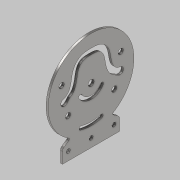
# Autodesk Inventor part: RR-PCSS-2021-W2M2MA2
Saved by Autodesk Inventor 2021 (Build 250183000, 183)
## iProperties
Created: 2021-10-12
Part Number: RR-PCSS-2021-W2M2MA2
Material: Stal nierdzewna
Document SubType Name: Konstrukcja blachowa
Designer: marci
Density: 8 g/cm^3
Sheet Metal Rule: Domyślny_mm
Appearance: Częściowo polerowana
Author: marci
Autodesk Inventor part; units mm, degrees
ref_plane "YZ Plane" through (0, 0, 0) normal (1, 0, 0) x (0, 1, 0)
ref_plane "XZ Plane" through (0, 0, 0) normal (0, 1, 0) x (-1, 0, 0)
ref_plane "XY Plane" through (0, 0, 0) normal (0, 0, 1) x (1, 0, 0)
sketch "Szkic1" plane through (0, 0, 0) normal (1, 0, 0) x (0, 1, 0)
  arc A0 (305.2016, 165.6304) -> (305.2016, 131.3696) centre (315.5238, 148.5) ccw
  arc A1 (307.7821, 161.3478) -> (305.2016, 165.6304) centre (306.4918, 163.4891) ccw
  arc A2 (307.7821, 161.3478) -> (307.7821, 135.6522) centre (315.5238, 148.5) ccw
  arc A3 (305.2016, 131.3696) -> (307.7821, 135.6522) centre (306.4918, 133.5109) ccw
  circle A4 centre (292.0124, 180.8607) radius 3.65
  circle A5 centre (333.1067, 189.9227) radius 3.65
  circle A6 centre (333.1067, 107.0773) radius 3.65
  circle A7 centre (292.0124, 116.1393) radius 3.65
  arc A8 (265.7342, 133.5) -> (270.5217, 134.9423) centre (268.128, 134.2212) ccw
  arc A9 (265.7342, 163.5) -> (265.7342, 133.5) centre (315.5238, 148.5) ccw
  arc A10 (270.5217, 162.0577) -> (265.7342, 163.5) centre (268.128, 162.7788) ccw
  arc A11 (270.5217, 162.0577) -> (270.5217, 134.9423) centre (315.5238, 148.5) ccw
  spline S0 degree 3 poles (357.7316, 148.5) (357.7316, 153.1999) (357.4798, 157.3219) (355.4595, 163.5199) (354.2505, 165.5182) (351.0648, 169.1973) (348.9327, 170.8743) (343.9224, 173.7031) (341.1419, 174.5841) (332.899, 176.2956) (327.9871, 176.7072) (321.7354, 179.3107) (319.9473, 180.4312) (317.422, 182.9628) (316.5959, 184.0618) (315.07, 186.6603) (315.3905, 188.1626) (314.1922, 189.4328) knots -9.163844 -9.163844 -9.163844 -9.163844 -7.753869 -7.753869 -6.746587 -6.746587 -5.59383 -5.59383 -4.201497 -4.201497 -2.238429 -2.238429 -1.297056 -1.297056 -0.700858 -0.700858 0 0 0 0
  line L0 (357.7316, 148.5) -> (357.7316, 153.1999) construction
  line L1 (357.7316, 153.1999) -> (357.4798, 157.3219) construction
  line L2 (357.4798, 157.3219) -> (355.4595, 163.5199) construction
  line L3 (355.4595, 163.5199) -> (354.2505, 165.5182) construction
  line L4 (354.2505, 165.5182) -> (351.0648, 169.1973) construction
  line L5 (351.0648, 169.1973) -> (348.9327, 170.8743) construction
  line L6 (348.9327, 170.8743) -> (343.9224, 173.7031) construction
  line L7 (343.9224, 173.7031) -> (341.1419, 174.5841) construction
  line L8 (341.1419, 174.5841) -> (332.899, 176.2956) construction
  line L9 (332.899, 176.2956) -> (327.9871, 176.7072) construction
  line L10 (327.9871, 176.7072) -> (321.7354, 179.3107) construction
  line L11 (321.7354, 179.3107) -> (319.9473, 180.4312) construction
  line L12 (319.9473, 180.4312) -> (317.422, 182.9628) construction
  line L13 (317.422, 182.9628) -> (316.5959, 184.0618) construction
  line L14 (316.5959, 184.0618) -> (315.07, 186.6603) construction
  line L15 (315.07, 186.6603) -> (315.3905, 188.1626) construction
  line L16 (315.3905, 188.1626) -> (314.1922, 189.4328) construction
  spline S1 degree 3 poles (314.7636, 107.2836) (315.1895, 110.0737) (316.0926, 112.3675) (318.7997, 115.5706) (320.2643, 116.7452) (323.9682, 118.7687) (326.1559, 119.4488) (333.914, 121.2316) (340.1639, 121.52) (348.3717, 125.6837) (350.9092, 127.5926) (354.3009, 131.5638) (355.4987, 133.5584) (357.4842, 139.7513) (357.7316, 143.8417) (357.7316, 148.5) knots -7.999364 -7.999364 -7.999364 -7.999364 -7.089801 -7.089801 -6.306276 -6.306276 -5.390174 -5.390174 -3.08524 -3.08524 -1.97401 -1.97401 -1.144907 -1.144907 0 0 0 0
  line L17 (314.7636, 107.2836) -> (315.1895, 110.0737) construction
  line L18 (315.1895, 110.0737) -> (316.0926, 112.3675) construction
  line L19 (316.0926, 112.3675) -> (318.7997, 115.5706) construction
  line L20 (318.7997, 115.5706) -> (320.2643, 116.7452) construction
  line L21 (320.2643, 116.7452) -> (323.9682, 118.7687) construction
  line L22 (323.9682, 118.7687) -> (326.1559, 119.4488) construction
  line L23 (326.1559, 119.4488) -> (333.914, 121.2316) construction
  line L24 (333.914, 121.2316) -> (340.1639, 121.52) construction
  line L25 (340.1639, 121.52) -> (348.3717, 125.6837) construction
  line L26 (348.3717, 125.6837) -> (350.9092, 127.5926) construction
  line L27 (350.9092, 127.5926) -> (354.3009, 131.5638) construction
  line L28 (354.3009, 131.5638) -> (355.4987, 133.5584) construction
  line L29 (355.4987, 133.5584) -> (357.4842, 139.7513) construction
  line L30 (357.4842, 139.7513) -> (357.7316, 143.8417) construction
  line L31 (357.7316, 143.8417) -> (357.7316, 148.5) construction
  arc A12 (305.7086, 110.17) -> (314.7636, 107.2836) centre (310.0075, 108.0096) ccw
  spline S2 degree 3 poles (349.7316, 148.5) (349.7316, 144.263) (349.5035, 141.031) (348.232, 137.1168) (347.6126, 136.0385) (345.6418, 133.7599) (344.2226, 132.6472) (340.9385, 130.8081) (339.0257, 130.1351) (331.2404, 128.5496) (325.7415, 128.0559) (318.2028, 124.8703) (315.3125, 123.2792) (311.2172, 119.1288) (309.9943, 117.5052) (307.7133, 113.5974) (306.4514, 111.648) (305.7086, 110.17) knots -6.764215 -6.764215 -6.764215 -6.764215 -5.493128 -5.493128 -4.764431 -4.764431 -3.885162 -3.885162 -2.898584 -2.898584 -1.437025 -1.437025 -0.780111 -0.780111 -0.427062 -0.427062 0 0 0 0
  line L32 (349.7316, 148.5) -> (349.7316, 144.263) construction
  line L33 (349.7316, 144.263) -> (349.5035, 141.031) construction
  line L34 (349.5035, 141.031) -> (348.232, 137.1168) construction
  line L35 (348.232, 137.1168) -> (347.6126, 136.0385) construction
  line L36 (347.6126, 136.0385) -> (345.6418, 133.7599) construction
  line L37 (345.6418, 133.7599) -> (344.2226, 132.6472) construction
  line L38 (344.2226, 132.6472) -> (340.9385, 130.8081) construction
  line L39 (340.9385, 130.8081) -> (339.0257, 130.1351) construction
  line L40 (339.0257, 130.1351) -> (331.2404, 128.5496) construction
  line L41 (331.2404, 128.5496) -> (325.7415, 128.0559) construction
  line L42 (325.7415, 128.0559) -> (318.2028, 124.8703) construction
  line L43 (318.2028, 124.8703) -> (315.3125, 123.2792) construction
  line L44 (315.3125, 123.2792) -> (311.2172, 119.1288) construction
  line L45 (311.2172, 119.1288) -> (309.9943, 117.5052) construction
  line L46 (309.9943, 117.5052) -> (307.7133, 113.5974) construction
  line L47 (307.7133, 113.5974) -> (306.4514, 111.648) construction
  line L48 (306.4514, 111.648) -> (305.7086, 110.17) construction
  spline S3 degree 3 poles (305.9798, 187.099) (305.3527, 184.0453) (308.7468, 180.9276) (313.5871, 177.5597) (314.8029, 174.123) (320.8963, 170.7927) (323.757, 169.8973) (332.0444, 167.982) (337.6971, 167.6683) (343.529, 164.8366) (345.3172, 163.5919) (347.6017, 160.9896) (348.2119, 159.9056) (349.4982, 156.0549) (349.7316, 152.7861) (349.7316, 148.5) knots -3.192679 -3.192679 -3.192679 -3.192679 -2.291125 -2.291125 -1.878784 -1.878784 -1.540993 -1.540993 -0.855442 -0.855442 -0.570127 -0.570127 -0.370811 -0.370811 0 0 0 0
  line L49 (305.9798, 187.099) -> (305.3527, 184.0453) construction
  line L50 (305.3527, 184.0453) -> (308.7468, 180.9276) construction
  line L51 (308.7468, 180.9276) -> (313.5871, 177.5597) construction
  line L52 (313.5871, 177.5597) -> (314.8029, 174.123) construction
  line L53 (314.8029, 174.123) -> (320.8963, 170.7927) construction
  line L54 (320.8963, 170.7927) -> (323.757, 169.8973) construction
  line L55 (323.757, 169.8973) -> (332.0444, 167.982) construction
  line L56 (332.0444, 167.982) -> (337.6971, 167.6683) construction
  line L57 (337.6971, 167.6683) -> (343.529, 164.8366) construction
  line L58 (343.529, 164.8366) -> (345.3172, 163.5919) construction
  line L59 (345.3172, 163.5919) -> (347.6017, 160.9896) construction
  line L60 (347.6017, 160.9896) -> (348.2119, 159.9056) construction
  line L61 (348.2119, 159.9056) -> (349.4982, 156.0549) construction
  line L62 (349.4982, 156.0549) -> (349.7316, 152.7861) construction
  line L63 (349.7316, 152.7861) -> (349.7316, 148.5) construction
  arc A13 (314.1922, 189.4328) -> (305.9798, 187.099) centre (310.6926, 186.1312) ccw
  circle A14 centre (315.5238, 148.5) radius 4.15
  arc A15 (264, 117.7543) -> (264, 179.2457) centre (315.5238, 148.5) ccw
  line L64 (375.5238, 148.5) -> (375.5238, 88.5)
  line L65 (237, 148.5) -> (297, 148.5) construction
  line L66 (375.5238, 88.5) -> (237, 88.5)
  line L67 (237, 208.5) -> (375.5238, 208.5)
  line L68 (375.5238, 208.5) -> (375.5238, 88.5)
  line L69 (237, 148.5) -> (237, 188.5)
  line L70 (237, 148.5) -> (237, 108.5)
  line L71 (237, 188.5) -> (237, 208.5)
  line L72 (237, 108.5) -> (237, 88.5)
  line L73 (243, 169.1907) -> (243, 188.5)
  line L74 (243, 188.5) -> (252.4205, 188.5)
  line L75 (264, 179.2457) -> (263.7142, 179.1089)
  line L76 (261.2206, 179.7536) -> (256.495, 186.3979)
  arc A16 (256.495, 186.3979) -> (252.4205, 188.5) centre (252.4205, 183.5) ccw
  arc A17 (261.2206, 179.7536) -> (263.7142, 179.1089) centre (262.8505, 180.9127) ccw
  line L77 (264, 117.7543) -> (263.8601, 117.8366)
  line L78 (243, 130.1131) -> (243, 108.5)
  line L79 (243, 108.5) -> (252.4149, 108.5)
  line L80 (256.4946, 110.6092) -> (261.2139, 117.2693)
  arc A18 (263.8601, 117.8366) -> (261.2139, 117.2693) centre (262.8457, 116.113) ccw
  arc A19 (252.4149, 108.5) -> (256.4946, 110.6092) centre (252.4149, 113.5) ccw
  line L81 (243, 108.5) -> (237, 108.5)
  line L82 (243, 188.5) -> (237, 188.5)
  line L83 (243, 88.5) -> (243, 108.5)
  line L84 (243, 148.5) -> (243, 208.5)
  line L85 (243, 105.3032) -> (243, 108.5)
  line L86 (243, 188.5) -> (243, 194.6314)
  point P0 (0, 0)
  point P1 (235.8181, 152.9425)
  point P2 (226.82, 150.8873)
  point P3 (255, 188.5)
  point P4 (262.1961, 178.382)
  point P5 (262.2763, 118.7687)
  point P6 (255, 108.5)
  dimension "d0" = 60
  dimension "d1" = 60
  dimension "d3" = 40
  dimension "d4" = 40
  dimension "d14" = 40
  dimension "d15" = 12
  dimension "d16" = 2
  dimension "d17" = 5
  dimension "d18" = 2
  dimension "d19" = 2
  dimension "d20" = 40
  dimension "d21" = 12
  dimension "d22" = 2
  dimension "d23" = 5
  measures "d0" distance of L64.start L66.start
  measures "d1" distance of L65.start L67.start
  measures "d3" distance of L65.start L69.end
  measures "d4" distance of L65.start L70.end
  measures "d14" distance of L84.start L73.end
  measures "d15" distance of L73.end point (255, 188.5)
  measures "d16" distance of L75.start point (262.196, 178.382)
  measures "d17" radius of A16
  measures "d18" radius of A17
  measures "d19" distance of L77.start point (262.276, 118.769)
  measures "d20" distance of L84.start L78.end
  measures "d21" distance of L78.end point (255, 108.5)
  measures "d22" radius of A18
  measures "d23" radius of A19
extrude "Płyta2" add sketch "Szkic1" along normal blind 3 contours L77 A18 L80 A19 L79 L81 L70 L69 L82 L74 A16 L76 A17 L75 A15
sketch "Szkic2" plane through (0, 0, 0) normal (-1, 0, 0) x (0, 0, 1)
  point P0 (180.5, 249)
  point P1 (116.5, 249)
  point P2 (148.5, 249)
hole "Otwór1" at (0, 249, 180.5) at (0, 249, 116.5) at (0, 249, 148.5) direction (1, 0, 0) diameter 5.5 end through all
equation "\"d24\" = Grubość"
equation "\"PromieńGięcia\" = Grubość"
equation "\"SzerokośćGięciaPodcięcia\" = Grubość"
equation "\"GłębokośćGięciaPodcięcia\" = 0.5 * Grubość"
equation "\"RozmiarPodcięciaNarożnika\" = 4 * Grubość"
equation "\"MinimalnaPozostałość\" = 2 * Grubość"
equation "\"PromieńPrzejścia\" = PromieńGięcia"
equation "\"Rozmiar_promienia_Jacobiego\" = PromieńGięcia"
equation "\"Wielk_odstępu\" = Grubość"
equation "\"Grubość\" = 3"
